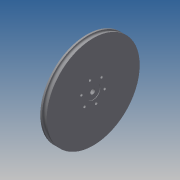
# Autodesk Inventor part: 7.25in Pully
Saved by Autodesk Inventor 2014 SP1 (Build 180222100, 222)
## iProperties
Created: 2014-01-29
Part Number: 7.25in Pully
Material: Generic
Document SubType Name: Modeling
Designer: Pradhan Alexander
Density: 1 g/cm^3
Appearance: Default
Author: Pradhan Alexander
Autodesk Inventor part; units mm, degrees
ref_plane "YZ Plane" through (0, 0, 0) normal (1, 0, 0) x (0, 1, 0)
ref_plane "XZ Plane" through (0, 0, 0) normal (0, 1, 0) x (-1, 0, 0)
ref_plane "XY Plane" through (0, 0, 0) normal (0, 0, 1) x (1, 0, 0)
sketch "Sketch1" plane through (0, 0, 0) normal (0, 0, 1) x (1, 0, 0)
  line L0 (-10.0445, -59.5143) -> (2.6555, -59.5143)
  line L1 (2.6555, -59.5143) -> (2.6555, 32.5607)
  line L2 (-10.0445, -59.5143) -> (-10.0445, 32.5607)
  line L3 (2.6555, 32.5607) -> (-0.5195, 32.5607)
  line L4 (-6.8695, 32.5607) -> (-10.0445, 32.5607)
  line L5 (-6.8695, 32.5607) -> (-6.8695, 32.1797)
  line L6 (-0.5195, 32.5607) -> (-0.5195, 32.1797)
  arc A0 (-6.8695, 32.1797) -> (-0.5195, 32.1797) centre (-3.6945, 32.1797) ccw
  point P0 (-8.457, 32.5607)
  point P1 (1.068, 32.5607)
  dimension "d0" = 12.7
  dimension "d3" = 92.075
  dimension "d4" = 0.381
  constraints: 14 end point, 3 equal length, 3 perpendicular, 2 midpoint, 2 point on circle, 2 tangent, 1 centre point, 1 horizontal, 1 horizontal alignment, 1 parallel
  measures "d0" distance between parallel lines of L1 L2
  measures "d3" distance of L0.start L2.end
  measures "d4" distance of L4.start L5.end
revolve "Revolution1" add sketch "Sketch1" angle 360 about axis through (-10.0445, -59.5143, 0) along (1, 0, 0)
sketch "Sketch2" plane through (2.6555, -59.5143, 0) normal (1, 0, 0) x (0, 0, -1)
  circle A0 centre (0, 0) radius 92.075 projected
  circle A1 centre (0, 0) radius 14.1224
  dimension "d6" = 28.2448
  constraints: 1 centre point, 1 coincident
  measures "d6" diameter of A1
extrude "Extrusion1" cut sketch "Sketch2" against normal blind 0.889 contours A1
sketch "Sketch3" plane through (1.7665, -59.5143, 0) normal (1, 0, 0) x (0, 0, -1)
  circle A0 centre (0, 0) radius 14.1224 projected
  constraints: 1 coincident
hole "Hole1" at (1.7665, -59.5143, 0) direction (-1, 0, 0) diameter 9.525 end through all
sketch "Sketch4" plane through (2.6555, -59.5143, 0) normal (1, 0, 0) x (0, 0, -1)
  circle A0 centre (16.847, 16.847) radius 2.54
  circle A1 centre (0, 0) radius 4.7625 projected
  line L0 (0, 0) -> (16.847, 16.847)
  dimension "d18" = 23.8252
  dimension "d24" = 5.08
  constraints: 2 end point, 1 centre point
  measures "d18" distance of L0.start L0.end
  measures "d24" diameter of A0
extrude "Extrusion2" cut sketch "Sketch4" against normal blind 10160 contours A0
pattern_circular "Circular Pattern1" count 6 over 360 about axis through (-258.9705, -59.5143, 0) along (1, 0, 0) of "Extrusion2"
body "Solid1"
